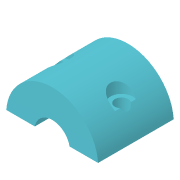
# Autodesk Inventor part: clamp
Saved by Autodesk Inventor 2018 (Build 220112000, 112)
## iProperties
Created: 2019-04-20
Part Number: clamp
Material: Generic
Document SubType Name: Modeling
Designer: amink
Density: 1 g/cm^3
Appearance: Default
Author: amink
Autodesk Inventor part; units mm, degrees
ref_plane "YZ Plane" through (0, 0, 0) normal (1, 0, 0) x (0, 1, 0)
ref_plane "XZ Plane" through (0, 0, 0) normal (0, 1, 0) x (-1, 0, 0)
ref_plane "XY Plane" through (0, 0, 0) normal (0, 0, 1) x (1, 0, 0)
sketch "Sketch1" plane through (0, 0, 0) normal (0, 0, 1) x (1, 0, 0)
  arc A0 (8.2335, 0.595) -> (-8.2335, 0.595) centre (0, 0) ccw
  arc A1 (3.1187, 0.595) -> (-3.1187, 0.595) centre (0, 0) ccw
  line L0 (-9.3675, 0.595) -> (10.1432, 0.595)
  line L1 (10.1432, 0.595) -> (10.1432, -0.595)
  line L2 (10.1432, -0.595) -> (-9.3675, -0.595)
  line L3 (-9.3675, -0.595) -> (-9.3675, 0.595)
  dimension "d0" = 16.51
  dimension "d1" = 6.35
  dimension "d2" = 1.19
  dimension "d3" = 0.595
  constraints: 8 end point, 4 point on circle, 4 point on line, 2 centre point, 2 coincident, 2 parallel, 1 horizontal, 1 perpendicular
  measures "d0" diameter of A0
  measures "d1" diameter of A1
  measures "d2" distance between parallel lines of L2 L0
  measures "d3" distance from line of point (0, 0) L2
extrude "Extrusion1" add sketch "Sketch1" along normal blind 13.573 contours L0 A1 A0
ref_plane "Work Plane2" through (0, 8.255, 0) normal (0, -1, 0) x (1, 0, 0)
ref_plane "Work Plane1" through (-8.2335, 8.85, 0) normal (0, -1, 0) x (1, 0, 0)
sketch "Sketch2" plane through (0, 8.255, 0) normal (0, -1, 0) x (1, 0, 0)
  circle A0 centre (-5.6761, 6.7865) radius 1.2
  line L0 (0, 0) -> (0, 16.3)
  line L1 (-3.1187, 0) -> (-3.1187, 13.573) projected
  line L2 (-8.2335, 0) -> (-8.2335, 13.573) projected
  line L3 (8.2335, 0) -> (-8.2335, 0) projected
  line L4 (8.2335, 13.573) -> (-8.2335, 13.573) projected
  circle A1 centre (5.6761, 6.7865) radius 1.2
  dimension "d7" = 2.4
  dimension "d8" = 5.1148
  dimension "d9" = 2.5574
  dimension "d10" = 13.573
  dimension "d11" = 6.7865
  constraints: 2 centre point, 2 end point, 1 symmetric about line, 1 vertical, 1 other
  measures "d7" diameter of A0
  measures "d8" distance between parallel lines of L1 L2
  measures "d9" distance from line of L1 A0.centre
  measures "d10" distance between parallel lines of L3 L4
  measures "d11" distance from line of L3 A0.centre
extrude "Extrusion2" cut sketch "Sketch2" along normal blind 25.4 contours A0 | A1
sketch "Sketch3" plane through (0, 8.255, 0) normal (0, -1, 0) x (1, 0, 0)
  circle A0 centre (-5.6761, 6.7865) radius 1.2 projected
  circle A1 centre (-5.6761, 6.7865) radius 2
  point P0 (0, 0)
  dimension "d14" = 4
  constraints: 1 centre point, 1 coincident
  measures "d14" diameter of A1
extrude "Extrusion3" cut sketch "Sketch3" along normal blind 3
mirror "Mirror1" about plane through (0, 0, 0) normal (1, 0, 0) of "Extrusion3"
equation "\"d3\" = 0.5 * d2"
equation "\"d9\" = 0.5 * d8"
equation "\"d11\" = 0.5 * d10"
body "Solid1"
